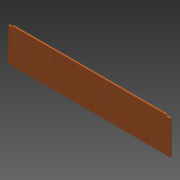
# Autodesk Inventor part: front-plate
Saved by Autodesk Inventor 2013 (Build 170138000, 138)
## iProperties
Created: 2013-05-01
Part Number: front-plate
Material: Wood (Cherry)
Document SubType Name: Modeling
Designer: Chris
Density: 1 g/cm^3
Author: Chris
Autodesk Inventor part; units mm, degrees
ref_plane "YZ Plane" through (0, 0, 0) normal (1, 0, 0) x (0, 1, 0)
ref_plane "XZ Plane" through (0, 0, 0) normal (0, 1, 0) x (-1, 0, 0)
ref_plane "XY Plane" through (0, 0, 0) normal (0, 0, 1) x (1, 0, 0)
sketch "Sketch1" plane through (0, 0, 0) normal (0, 0, 1) x (1, 0, 0)
  line L0 (0, 0) -> (1473.2, 0)
  line L1 (1473.2, 0) -> (1473.2, 304.8)
  line L2 (1473.2, 304.8) -> (0, 304.8)
  line L3 (0, 304.8) -> (0, 0)
  line L4 (38.1, 304.8) -> (1435.1, 304.8)
  line L5 (1435.1, 304.8) -> (1435.1, 317.5)
  line L6 (1435.1, 317.5) -> (38.1, 317.5)
  line L7 (38.1, 317.5) -> (38.1, 304.8)
  dimension "d0" = 1473.2
  dimension "d1" = 304.8
  dimension "d4" = 12.7
  dimension "d5" = 38.1
  dimension "d6" = 38.1
  constraints: 16 end point, 4 parallel, 2 horizontal, 2 perpendicular, 1 point on line
  measures "d0" distance of L2.end L1.end
  measures "d1" distance of L1.end L0.end
  measures "d4" distance of L5.end L4.end
  measures "d5" distance between parallel lines of L3 L7
  measures "d6" distance between parallel lines of L1 L5
extrude "Extrusion1" add sketch "Sketch1" along normal blind 12.7
equation "\"d6\" = d5"
body "Solid1"
